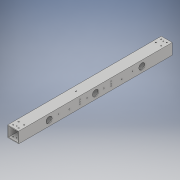
# Autodesk Inventor part: 2x2 26in
Saved by Autodesk Inventor 2019 (Build 230136000, 136)
## iProperties
Created: 2018-11-11
Part Number: 2x2 26in
Material: Generic
Document SubType Name: Modeling
Designer: maste
Density: 1 g/cm^3
Appearance: Default
Author: maste
Autodesk Inventor part; units mm, degrees
ref_plane "YZ Plane" through (0, 0, 0) normal (1, 0, 0) x (0, 1, 0)
ref_plane "XZ Plane" through (0, 0, 0) normal (0, 1, 0) x (-1, 0, 0)
ref_plane "XY Plane" through (0, 0, 0) normal (0, 0, 1) x (1, 0, 0)
sketch "Sketch1" plane through (0, 0, 0) normal (0, 0, 1) x (1, 0, 0)
  line L0 (0, 0) -> (50.8, 0)
  line L1 (50.8, 0) -> (50.8, 50.8)
  line L2 (50.8, 50.8) -> (0, 50.8)
  line L3 (0, 50.8) -> (0, 0)
  dimension "d0" = 50.8
  dimension "d1" = 50.8
  constraints: 8 end point, 2 parallel, 1 horizontal, 1 perpendicular
  measures "d0" distance of L2.end L1.end
  measures "d1" distance of L1.end L0.end
extrude "Extrusion1" add sketch "Sketch1" along normal blind 660.4
shell "Shell2" thickness 3.175 removed faces 2 at (16.9333, 33.8667, 660.4) at (16.9333, 33.8667, 0)
sketch "Sketch2" plane through (50.8, 0, 0) normal (1, 0, 0) x (0, 0, -1)
  line L0 (0, 3.175) -> (0, 47.625) projected
  line L1 (0, 25.4) -> (-115.189, 25.4)
  circle A0 centre (-115.189, 25.4) radius 14.2875
  line L2 (0, 50.8) -> (-660.4, 50.8) projected
  circle A1 centre (-545.211, 25.4) radius 14.2875
  circle A2 centre (-330.2, 25.4) radius 14.2875
  line L3 (0, 0) -> (-660.4, 0) projected
  line L4 (-330.2, 0) -> (-402.463, 0)
  circle A3 centre (-402.463, 26.9875) radius 2.54
  circle A4 centre (-402.463, 17.4625) radius 2.54
  circle A5 centre (-402.463, 36.5125) radius 2.54
  circle A6 centre (-257.937, 26.9875) radius 2.54
  circle A7 centre (-257.937, 17.4625) radius 2.54
  circle A8 centre (-257.937, 36.5125) radius 2.54
  dimension "d6" = 115.189
  dimension "d7" = 28.575
  dimension "d8" = 28.575
  dimension "d9" = 72.263
  dimension "d11" = 5.08
  constraints: 9 centre point, 4 end point, 2 midpoint, 1 coincident, 1 horizontal, 1 point on line
  measures "d6" distance of L1.start L1.end
  measures "d7" diameter of A0
  measures "d8" diameter of A2
  measures "d9" distance of L4.start L4.end
  measures "d11" diameter of A3
extrude "Extrusion2" cut sketch "Sketch2" against normal blind 660.4
sketch "Sketch3" plane through (0, 50.8, 0) normal (0, 1, 0) x (1, 0, 0)
  line L0 (21.4993, -395.7691) -> (21.4993, -389.053) construction
  line L1 (21.4993, -389.053) -> (25.4565, -389.053) construction
  line L2 (25.4565, -389.053) -> (25.4565, -395.7691) construction
  line L3 (25.4565, -395.7691) -> (21.4993, -395.7691) construction
  spline S0 degree 2 poles (21.9802, -393.2019) (21.9802, -393.3412) (21.9565, -393.6328) knots 0 0 0 1 1 1
  spline S1 degree 2 poles (21.9565, -393.6328) (21.9355, -393.914) (21.9381, -394.0611) knots 0 0 0 1 1 1
  line L4 (21.9381, -394.0611) -> (21.9381, -394.1951)
  spline S2 degree 2 poles (21.9381, -394.1951) (22.1983, -394.1899) (22.7842, -394.1452) knots 0 0 0 1 1 1
  spline S3 degree 2 poles (22.7842, -394.1452) (23.3281, -394.1032) (23.6303, -394.1032) knots 0 0 0 1 1 1
  spline S4 degree 2 poles (23.6303, -394.1032) (23.696, -394.1032) (23.964, -394.0769) (24.0323, -394.0769) knots 0 0 0 1 2 2 2
  spline S5 degree 2 poles (24.0323, -394.0769) (24.1584, -394.0769) (24.253, -394.1189) knots 0 0 0 1 1 1
  spline S6 degree 2 poles (24.253, -394.1189) (24.3765, -394.1715) (24.3765, -394.2819) knots 0 0 0 1 1 1
  spline S7 degree 2 poles (24.3765, -394.2819) (24.3765, -394.3581) (24.2714, -394.4789) (24.1873, -394.4789) knots 0 0 0 1 2 2 2
  spline S8 degree 2 poles (24.1873, -394.4789) (24.1584, -394.4789) (24.0455, -394.4605) (24.0192, -394.4605) knots 0 0 0 1 2 2 2
  spline S9 degree 2 poles (24.0192, -394.4605) (23.9246, -394.4605) (23.5567, -394.4842) (23.4621, -394.4842) knots 0 0 0 1 2 2 2
  spline S10 degree 2 poles (23.4621, -394.4842) (23.1915, -394.4842) (22.7028, -394.5288) knots 0 0 0 1 1 1
  spline S11 degree 2 poles (22.7028, -394.5288) (22.1772, -394.5735) (21.946, -394.5788) knots 0 0 0 1 1 1
  line L5 (21.946, -394.5788) -> (21.9486, -394.7496)
  spline S12 degree 2 poles (21.9486, -394.7496) (21.9486, -395.1621) (21.8882, -395.3986) knots 0 0 0 1 1 1
  spline S13 degree 2 poles (21.8882, -395.3986) (21.8488, -395.551) (21.7017, -395.551) knots 0 0 0 1 1 1
  spline S14 degree 2 poles (21.7017, -395.551) (21.6228, -395.551) (21.565, -395.5011) knots 0 0 0 1 1 1
  spline S15 degree 2 poles (21.565, -395.5011) (21.4993, -395.4459) (21.5046, -395.3565) knots 0 0 0 1 1 1
  spline S16 degree 2 poles (21.5046, -395.3565) (21.5072, -395.2908) (21.5387, -395.0544) knots 0 0 0 1 1 1
  spline S17 degree 2 poles (21.5387, -395.0544) (21.5624, -394.8678) (21.5624, -394.7496) knots 0 0 0 1 1 1
  spline S18 degree 2 poles (21.5624, -394.7496) (21.5624, -394.6366) (21.5519, -394.1767) (21.5519, -394.0638) knots 0 0 0 1 2 2 2
  spline S19 degree 2 poles (21.5519, -394.0638) (21.5519, -393.9192) (21.5939, -393.3491) (21.5939, -393.2019) knots 0 0 0 1 2 2 2
  spline S20 degree 2 poles (21.5939, -393.2019) (21.5939, -393.1231) (21.7043, -393.0127) (21.7884, -393.0127) knots 0 0 0 1 2 2 2
  spline S21 degree 2 poles (21.7884, -393.0127) (21.8672, -393.0127) (21.9802, -393.1231) (21.9802, -393.2019) knots 0 0 0 1 2 2 2
  spline S22 degree 2 poles (24.4711, -392.1745) (24.4711, -392.4898) (24.2373, -392.7184) knots 0 0 0 1 1 1
  spline S23 degree 2 poles (24.2373, -392.7184) (23.9771, -392.9733) (23.5383, -392.9865) knots 0 0 0 1 1 1
  spline S24 degree 2 poles (23.5383, -392.9865) (23.1127, -392.997) (22.7895, -392.771) knots 0 0 0 1 1 1
  spline S25 degree 2 poles (22.7895, -392.771) (22.4058, -392.5082) (22.4058, -392.0379) knots 0 0 0 1 1 1
  spline S26 degree 2 poles (22.4058, -392.0379) (22.4058, -391.6595) (22.7501, -391.4677) knots 0 0 0 1 1 1
  spline S27 degree 2 poles (22.7501, -391.4677) (23.0286, -391.3127) (23.4227, -391.3179) knots 0 0 0 1 1 1
  spline S28 degree 2 poles (23.4227, -391.3179) (23.8405, -391.3232) (24.1348, -391.536) knots 0 0 0 1 1 1
  spline S29 degree 2 poles (24.1348, -391.536) (24.4711, -391.7778) (24.4711, -392.1745) knots 0 0 0 1 1 1
  spline S30 degree 2 poles (22.7895, -392.0615) (22.7868, -392.3374) (23.0522, -392.4925) knots 0 0 0 1 1 1
  spline S31 degree 2 poles (23.0522, -392.4925) (23.2651, -392.616) (23.5383, -392.616) knots 0 0 0 1 1 1
  spline S32 degree 2 poles (23.5383, -392.616) (23.8116, -392.616) (23.964, -392.4662) knots 0 0 0 1 1 1
  spline S33 degree 2 poles (23.964, -392.4662) (24.0901, -392.3427) (24.0901, -392.1745) knots 0 0 0 1 1 1
  spline S34 degree 2 poles (24.0901, -392.1745) (24.0901, -391.9775) (23.9482, -391.8382) knots 0 0 0 1 1 1
  spline S35 degree 2 poles (23.9482, -391.8382) (23.788, -391.6779) (23.5199, -391.6674) knots 0 0 0 1 1 1
  spline S36 degree 2 poles (23.5199, -391.6674) (22.7921, -391.6411) (22.7895, -392.0615) knots 0 0 0 1 1 1
  spline S37 degree 2 poles (24.4265, -390.0541) (24.4265, -390.2433) (24.366, -390.4719) knots 0 0 0 1 1 1
  line L6 (24.366, -390.4719) -> (25.2673, -390.4745)
  spline S38 degree 2 poles (25.2673, -390.4745) (25.3514, -390.4745) (25.4565, -390.577) (25.4565, -390.6584) knots 0 0 0 1 2 2 2
  spline S39 degree 2 poles (25.4565, -390.6584) (25.4565, -390.7399) (25.3514, -390.8423) (25.2673, -390.8423) knots 0 0 0 1 2 2 2
  line L7 (25.2673, -390.8423) -> (24.5132, -390.8371)
  line L8 (24.5132, -390.8371) -> (23.7617, -390.8371)
  spline S40 degree 2 poles (23.7617, -390.8371) (23.3491, -390.8423) (23.0102, -390.866) knots 0 0 0 1 1 1
  line L9 (23.0102, -390.866) -> (22.6266, -390.8949)
  spline S41 degree 2 poles (22.6266, -390.8949) (22.4926, -390.8949) (22.4006, -390.845) knots 0 0 0 1 1 1
  spline S42 degree 2 poles (22.4006, -390.845) (22.2902, -390.7898) (22.2902, -390.6794) knots 0 0 0 1 1 1
  spline S43 degree 2 poles (22.2902, -390.6794) (22.2902, -390.6059) (22.3927, -390.506) (22.4689, -390.506) knots 0 0 0 1 2 2 2
  spline S44 degree 2 poles (22.4689, -390.506) (22.4873, -390.506) (22.532, -390.5113) knots 0 0 0 1 1 1
  spline S45 degree 2 poles (22.532, -390.5113) (22.5898, -390.5218) (22.6397, -390.5244) knots 0 0 0 1 1 1
  spline S46 degree 2 poles (22.6397, -390.5244) (22.5267, -390.3615) (22.4164, -390.0593) (22.4164, -389.9227) knots 0 0 0 1 2 2 2
  spline S47 degree 2 poles (22.4164, -389.9227) (22.4164, -389.5364) (22.7579, -389.3578) knots 0 0 0 1 1 1
  spline S48 degree 2 poles (22.7579, -389.3578) (23.0312, -389.2159) (23.4779, -389.2159) knots 0 0 0 1 1 1
  spline S49 degree 2 poles (23.4779, -389.2159) (23.8852, -389.2159) (24.1479, -389.434) knots 0 0 0 1 1 1
  spline S50 degree 2 poles (24.1479, -389.434) (24.4265, -389.6678) (24.4265, -390.0541) knots 0 0 0 1 1 1
  spline S51 degree 2 poles (22.7921, -389.9253) (22.7921, -390.0987) (22.8683, -390.238) knots 0 0 0 1 1 1
  spline S52 degree 2 poles (22.8683, -390.238) (22.9235, -390.3378) (23.068, -390.4902) knots 0 0 0 1 1 1
  spline S53 degree 2 poles (23.068, -390.4902) (23.4963, -390.4666) (23.9693, -390.4666) knots 0 0 0 1 1 1
  spline S54 degree 2 poles (23.9693, -390.4666) (24.0481, -390.2616) (24.0481, -390.0541) knots 0 0 0 1 1 1
  spline S55 degree 2 poles (24.0481, -390.0541) (24.0481, -389.8176) (23.872, -389.6941) knots 0 0 0 1 1 1
  spline S56 degree 2 poles (23.872, -389.6941) (23.7196, -389.5864) (23.4779, -389.5864) knots 0 0 0 1 1 1
  spline S57 degree 2 poles (23.4779, -389.5864) (23.1337, -389.5864) (22.7921, -389.7545) (22.7921, -389.9253) knots 0 0 0 1 2 2 2
  point P0 (0, 0)
  constraints: 2 other
emboss "Emboss1" sketch "Sketch3" operation cut depth 0.254 direction (0, -1, 0)
sketch "Sketch5" plane through (0, 0, 0) normal (-1, 0, 0) x (0, 0, 1)
  circle A0 centre (330.2, 25.4) radius 14.2875 projected
  line L0 (330.2, 25.4) -> (368.3, 25.4)
  line L1 (330.2, 25.4) -> (292.1, 25.4)
  circle A1 centre (292.1, 25.4) radius 2.54
  circle A2 centre (368.3, 25.4) radius 2.54
  point P0 (0, 0)
  dimension "d18" = 38.1
  dimension "d19" = 38.1
  dimension "d20" = 5.08
  dimension "d21" = 5.08
  constraints: 4 end point, 2 centre point, 2 coincident, 2 horizontal
  measures "d18" distance of L0.start L0.end
  measures "d19" distance of L0.start L1.end
  measures "d20" diameter of A1
  measures "d21" diameter of A2
extrude "Extrusion3" cut sketch "Sketch5" against normal blind 660.4 contours A1 | A2
sketch "Sketch6" plane through (0, 0, 660.4) normal (0, 0, 1) x (1, 0, 0)
  line L0 (0, 0) -> (50.8, 0) projected
  line L1 (0, 0) -> (50.8, 0)
  line L2 (50.8, 0) -> (50.8, 50.8)
  line L3 (50.8, 50.8) -> (0, 50.8)
  line L4 (0, 50.8) -> (0, 0)
  line L5 (3.175, 3.175) -> (47.625, 3.175)
  line L6 (47.625, 3.175) -> (47.625, 47.625)
  line L7 (47.625, 47.625) -> (3.175, 47.625)
  line L8 (3.175, 47.625) -> (3.175, 3.175)
  constraints: 16 end point, 4 parallel, 2 horizontal, 2 perpendicular
extrude "Extrusion4" add sketch "Sketch6" along normal blind 25.4
sketch "Sketch7" plane through (0, 0, 0) normal (0, 0, -1) x (-1, 0, 0)
  line L0 (-50.8, 0) -> (-50.8, 50.8) projected
  line L1 (0, 0) -> (-50.8, 0)
  line L2 (-50.8, 0) -> (-50.8, 50.8)
  line L3 (-50.8, 50.8) -> (0, 50.8)
  line L4 (0, 50.8) -> (0, 0)
  line L5 (-3.175, 47.625) -> (-3.175, 3.175) projected
  line L6 (-47.625, 3.175) -> (-47.625, 47.625) projected
  line L7 (-3.175, 3.175) -> (-47.625, 3.175)
  line L8 (-47.625, 3.175) -> (-47.625, 47.625)
  line L9 (-47.625, 47.625) -> (-3.175, 47.625)
  line L10 (-3.175, 47.625) -> (-3.175, 3.175)
  constraints: 16 end point, 4 parallel, 2 horizontal, 2 perpendicular
extrude "Extrusion5" add sketch "Sketch7" along normal blind 25.4
sketch "Sketch8" plane through (0, 50.8, 685.8) normal (0, 1, 0) x (1, 0, 0)
  line L0 (0, 711.2) -> (50.8, 711.2) projected
  line L1 (0, 711.2) -> (50.8, 711.2)
  line L2 (50.8, 711.2) -> (50.8, 660.4)
  line L3 (50.8, 660.4) -> (0, 660.4)
  line L4 (0, 660.4) -> (0, 711.2)
  line L5 (38.1, 673.1) -> (38.1, 698.5)
  line L6 (38.1, 698.5) -> (12.7, 698.5)
  line L7 (12.7, 698.5) -> (12.7, 673.1)
  line L8 (12.7, 673.1) -> (38.1, 673.1)
  circle A0 centre (12.7, 698.5) radius 2.54
  circle A1 centre (38.1, 698.5) radius 2.54
  circle A2 centre (38.1, 673.1) radius 2.54
  circle A3 centre (12.7, 673.1) radius 2.54
  line L9 (0, 0) -> (0, 711.2) projected
  line L10 (0, 355.6) -> (50.8, 355.6)
  line L11 (0, 0) -> (50.8, 0)
  line L12 (0, 0) -> (50.8, 0)
  line L13 (50.8, 0) -> (50.8, 50.8)
  line L14 (50.8, 50.8) -> (0, 50.8)
  line L15 (0, 50.8) -> (0, 0)
  line L16 (38.1, 38.1) -> (38.1, 12.7)
  line L17 (38.1, 12.7) -> (12.7, 12.7)
  line L18 (12.7, 12.7) -> (12.7, 38.1)
  line L19 (12.7, 38.1) -> (38.1, 38.1)
  circle A4 centre (12.7, 12.7) radius 2.54
  circle A5 centre (38.1, 12.7) radius 2.54
  circle A6 centre (38.1, 38.1) radius 2.54
  circle A7 centre (12.7, 38.1) radius 2.54
  line L20 (0, 711.2) -> (0, 0)
  point P0 (0, 685.8)
  point P1 (0, 25.4)
  dimension "d28" = 50.8
  dimension "d29" = 12.7
  dimension "d30" = 5.08
  dimension "d33" = 25.4
  constraints: 38 end point, 15 symmetric about line, 8 centre point, 8 coincident, 4 parallel, 2 horizontal, 2 perpendicular, 1 midpoint, 7 other
  measures "d28" distance of L2.end L3.end
  measures "d29" distance between parallel lines of L2 L5
  measures "d30" diameter of A0
  measures "d33" distance of L16.start L17.start
extrude "Extrusion6" cut sketch "Sketch8" against normal blind 76.2 contours L8 A2 L5 | L5 A2 L8 | A1 L6 L5 | L5 L6 A1 | A3 L7 L8 | L8 L7 A3 | A0 L7 L6 | L6 L7 A0 | L19 A6 L16 | L16 A6 L19 | A5 L17 L16 | L16 L17 A5 | A7 L18 L19 | L19 L18 A7 | A4 L18 L17 | L17 L18 A4
sketch "Sketch9" plane through (50.8, 0, 685.8) normal (1, 0, 0) x (0, 0, -1)
  line L0 (711.2, 0) -> (0, 0) projected
  line L1 (711.2, 0) -> (476.25, 0)
  line L2 (476.25, 0) -> (476.25, 20.6375)
  circle A0 centre (476.25, 20.6375) radius 2.54
  line L3 (711.2, 50.8) -> (0, 50.8) projected
  line L4 (355.6, 50.8) -> (355.6, 0)
  circle A1 centre (234.95, 20.6375) radius 2.54
  point P0 (685.8, 0)
  dimension "d34" = 234.95
  dimension "d35" = 20.6375
  dimension "d36" = 5.08
  constraints: 6 end point, 2 centre point, 2 midpoint, 1 coincident, 1 perpendicular, 1 point on line, 1 symmetric about line, 1 other
  measures "d34" distance of L0.start L1.end
  measures "d35" distance of L1.end L2.end
  measures "d36" diameter of A0
extrude "Extrusion7" cut sketch "Sketch9" against normal blind 76.2
sketch "Sketch10" plane through (0, 50.8, 685.8) normal (0, 1, 0) x (1, 0, 0)
  line L0 (0, 711.2) -> (50.8, 711.2) projected
  line L1 (25.4, 711.2) -> (25.4, 695.325)
  circle A0 centre (25.4, 695.325) radius 2.159
  line L2 (50.8, 0) -> (0, 0) projected
  line L3 (25.4, 0) -> (25.4, 15.875)
  circle A1 centre (25.4, 15.875) radius 2.159
  point P0 (0, 685.8)
  point P1 (38.1, 698.5)
  point P2 (12.7, 673.1)
  point P3 (12.7, 698.5)
  point P4 (38.1, 673.1)
  point P5 (38.1, 38.1)
  dimension "d42" = 15.875
  dimension "d43" = 15.875
  constraints: 4 end point, 2 centre point, 2 coincident, 2 midpoint, 2 vertical
  measures "d42" distance of L1.start L1.end
  measures "d43" distance of L3.start L3.end
extrude "Extrusion8" cut sketch "Sketch10" against normal blind 109.5375
sketch "Sketch11" plane through (50.8, 0, 685.8) normal (1, 0, 0) x (0, 0, -1)
  line L0 (711.2, 50.8) -> (0, 50.8) projected
  line L1 (570.6761, 50.8) -> (570.6761, 22.86)
  line L2 (570.6761, 22.86) -> (534.45, 27.1092)
  line L3 (534.45, 27.1092) -> (527.1348, 27.1092)
  circle A0 centre (527.1348, 27.1092) radius 2.0193
  line L4 (355.6, 50.8) -> (355.6, 0)
  circle A1 centre (184.0652, 27.1092) radius 2.0193
  point P0 (685.8, 0)
  dimension "d44" = 27.94
  dimension "d45" = 36.4744
  dimension "d46" = 83.31
  dimension "d47" = 7.3152
  dimension "d48" = 4.0386
  constraints: 8 end point, 2 centre point, 2 vertical, 1 coincident, 1 horizontal, 1 midpoint, 1 point on line, 1 symmetric about line, 1 other
  measures "d44" distance of L1.start L1.end
  measures "d45" distance of L1.end L2.end
  measures "d46" angle of L1 L2
  measures "d47" distance of L2.end L3.end
  measures "d48" diameter of A0
extrude "Extrusion9" cut sketch "Sketch11" against normal blind 109.5375
body "Solid1"
